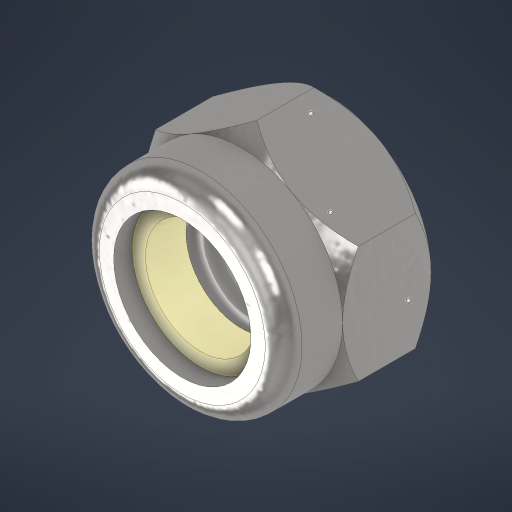
# Autodesk Inventor part: M1.6
Saved by Autodesk Inventor 2023.1 (Build 271208000, 208)
## iProperties
Created: 2022-08-21
Part Number: M1.6
Material: Steel, Galvanized
Document SubType Name: Modeling
Designer: ABL
Density: 7.85 g/cm^3
Appearance: Galvanized
Author: ABL
Autodesk Inventor part; units mm, degrees
ref_plane "YZ Plane" through (0, 0, 0) normal (1, 0, 0) x (0, 1, 0)
ref_plane "XZ Plane" through (0, 0, 0) normal (0, 1, 0) x (-1, 0, 0)
ref_plane "XY Plane" through (0, 0, 0) normal (0, 0, 1) x (1, 0, 0)
sketch "Sketch1" plane through (0, 0, 0) normal (0, 0, 1) x (1, 0, 0)
  line L0 (0, 3.1754) -> (2.75, 1.5877)
  line L1 (2.75, 1.5877) -> (2.75, -1.5877)
  line L2 (2.75, -1.5877) -> (0, -3.1754)
  line L3 (0, -3.1754) -> (-2.75, -1.5877)
  line L4 (-2.75, -1.5877) -> (-2.75, 1.5877)
  line L5 (-2.75, 1.5877) -> (0, 3.1754)
  point P0 (0, 0)
  point P1 (0, 0)
  dimension "d0" = 5.5
  constraints: 12 end point, 1 coincident, 1 vertical, 13 other
  measures "d0" distance between parallel lines of L1 L4
extrude "Main Body" add sketch "Sketch1" along normal blind 2.4
sketch "Sketch2" plane through (0, 0, 2.4) normal (0, 0, 1) x (1, 0, 0)
  circle A0 centre (0, 0) radius 2.75
  line L0 (2.75, -1.5877) -> (2.75, 1.5877) construction
  point P0 (2.75, 0)
  constraints: 1 coincident, 1 horizontal alignment, 1 midpoint, 2 other
extrude "Front Taper" cut sketch "Sketch2" against normal up to surface (2.4 mm away) draft 45 keep common part
sketch "Sketch3" plane through (0, 0, 0) normal (0, 0, -1) x (-1, 0, 0)
  circle A0 centre (0, 0) radius 2.75
  line L0 (-2.75, -1.5877) -> (-2.75, 1.5877) projected
  point P0 (-2.75, 0)
  constraints: 1 coincident, 1 horizontal alignment, 1 midpoint, 2 other
extrude "Back Taper" cut sketch "Sketch3" against normal up to surface (2.4 mm away) draft 45 keep common part
sketch "Sketch4" plane through (0, 0, 2.4) normal (0, 0, 1) x (1, 0, 0)
  circle A0 centre (0, 0) radius 1.5
  dimension "d9" = 3
  constraints: 1 centre point, 1 coincident
  measures "d9" diameter of A0
extrude "Center Hole" cut sketch "Sketch4" against normal up to surface (2.4 mm away)
sketch "Sketch6" plane through (0, 0, 0) normal (0, 1, 0) x (-1, 0, 0)
  line L0 (-2.75, 0) -> (-2.75, 2.4) projected
  line L1 (-2.75, 2.4) -> (-1.5, 2.4) projected
  line L2 (-1.5, 0) -> (-2.75, 0) projected
  line L3 (2.75, 2.4) -> (2.75, 0) projected
  line L4 (2.75, 0) -> (1.5, 0) projected
  line L5 (1.5, 2.4) -> (2.75, 2.4) projected
  line L6 (1.5, 2.4) -> (1.8616, 2.4)
  line L7 (1.8616, 2.4) -> (1.8616, 3.5)
  line L8 (1.8616, 3.5) -> (1.5, 3.5)
  line L9 (1.5, 3.5) -> (1.5, 2.4)
  line L10 (1.8616, 2.4) -> (2.75, 2.4)
  line L11 (2.75, 2.4) -> (2.75, 4)
  line L12 (2.75, 4) -> (1.8616, 4)
  line L13 (1.8616, 4) -> (1.8616, 2.4)
  line L14 (0, -1.0258) -> (0, 4.8376) projected
  line L15 (-1.5, 2.4) -> (-1.5, 0) projected
  line L16 (1.5, 0) -> (1.5, 2.4) projected
  point P0 (0, 0)
  dimension "d35" = 0.3616
  dimension "d36" = 1.6
  dimension "d37" = 0.5
  constraints: 16 end point, 4 parallel, 2 horizontal, 2 perpendicular, 1 point on line
  measures "d35" distance of L8.end L7.end
  measures "d36" distance of L10.end L11.end
  measures "d37" distance between parallel lines of L12 L8
revolve "Locking Cap" add sketch "Sketch6" angle 360 about axis through (0, 0, -10) along (0, 0, 1) contours L5 L7 L13 L12 L11
fillet "Fillet1" radius 0.5 1 edges at (2.75, 0, 4)
revolve "Nylon Locking" add sketch "Sketch6" angle 360 about axis through (0, 0, -10) along (0, 0, 1) separate body contours L5 L9 L8 L7
thread "Thread1" size "M3x0.5" class "6H" standard "ANSI Metric M Profile" full length
sketch "Sketch5" plane through (0, 0, 0) normal (1, 0, 0) x (0, 1, 0)
  line L0 (-1.8259, 3.2833) -> (-1.5, 3.4714)
  line L1 (-1.5, 3.4714) -> (-1.5, 2.9714)
  line L2 (-1.5, 2.9714) -> (-1.8259, 3.1596)
  line L3 (-1.933, 3.2214) -> (-1.5, 3.2214) construction
  line L4 (-1.5, 2.4) -> (1.5, 2.4) construction
  arc A0 (-1.8259, 3.2833) -> (-1.8259, 3.1596) centre (-1.7902, 3.2214) ccw
  point P0 (0, 0)
  point P1 (-1.6443, 3.2214)
  point P2 (-1.8616, 3.2214)
  dimension "d14" = 0.5
  dimension "d15" = 0.5714
  dimension "d16" = 0
  dimension "d17" = 0.0714
  dimension "d33" = 0.3616
  constraints: 8 end point, 3 point on circle, 2 point on line, 2 tangent, 1 centre point, 1 horizontal, 1 midpoint, 7 other
  measures "d14" distance of L0.end L1.end
  measures "d15" distance from line of L4 L1.end
  measures "d16" distance from line of L4.start L1
  measures "d17" radius of A0
  measures "d33" distance of L3.end point (-1.862, 3.221)
coil "Coil1" [suppressed]
equation "\"d0\" = size"
equation "\"d1\" = sideHeight"
equation "\"d9\" = nominalDiameter"
equation "\"d35\" = d33"
equation "\"d36\" = lockingHeight"
equation "\"d37\" = threadPitch"
equation "\"d40\" = d37"
equation "\"d14\" = threadPitch"
equation "\"d15\" = 1.14286 * threadPitch"
equation "\"d17\" = 0.142857 * threadPitch"
equation "\"d18\" = threadPitch"
equation "\"d19\" = 1.57143 * sideHeight"
equation "\"size\" = 5.5"
equation "\"sideHeight\" = 2.4"
equation "\"nominalDiameter\" = 3"
equation "\"threadPitch\" = 0.5"
equation "\"thickness\" = 4"
equation "\"lockingHeight\" = thickness - sideHeight"
equation "\"d29\" = 0.5 * size - 0.5 * nominalDiameter - threadPitch"
